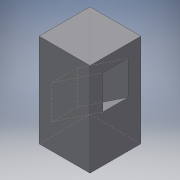
# Autodesk Inventor part: hollow monitor support (for assembly)
Saved by Autodesk Inventor 2016 (Build 200138000, 138)
## iProperties
Created: 2017-10-26
Part Number: hollow monitor support (for assembly)
Material: Generic
Document SubType Name: Modeling
Designer: student
Density: 1 g/cm^3
Appearance: Default
Author: student
Autodesk Inventor part; units mm, degrees
ref_plane "YZ Plane" through (0, 0, 0) normal (1, 0, 0) x (0, 1, 0)
ref_plane "XZ Plane" through (0, 0, 0) normal (0, 1, 0) x (-1, 0, 0)
ref_plane "XY Plane" through (0, 0, 0) normal (0, 0, 1) x (1, 0, 0)
sketch "Sketch1" plane through (0, 0, 0) normal (0, 0, 1) x (1, 0, 0)
  line L0 (-38.1, -69.85) -> (38.1, -69.85)
  line L1 (38.1, -69.85) -> (38.1, 69.85)
  line L2 (38.1, 69.85) -> (-38.1, 69.85)
  line L3 (-38.1, 69.85) -> (-38.1, -69.85)
  line L4 (38.1, 6.35) -> (-38.1, -57.15)
  line L5 (38.1, 57.15) -> (-38.1, -6.35)
  point P0 (0, 0)
  dimension "d0" = 139.7
  dimension "d1" = 76.2
  dimension "d2" = 76.2
  dimension "d3" = 12.7
  dimension "d5" = 12.7
  dimension "d12" = 76.2
  constraints: 12 end point, 4 point on line, 2 parallel, 1 horizontal, 1 perpendicular
  measures "d0" distance of L0.end L1.end
  measures "d1" distance of L0.start L0.end
  measures "d2" distance of L0.end L4.start
  measures "d3" distance of L0.start L4.end
  measures "d5" distance of L1.end L5.start
  measures "d12" distance from line of L2 L5.end
extrude "Extrusion1" add sketch "Sketch1" along normal blind 38.1 contours L3 L4 L1 L0 | L3 L2 L1 L5
sketch "Sketch2" plane through (0, 0, 38.1) normal (0, 0, 1) x (1, 0, 0)
  line L0 (-38.1, 69.85) -> (-38.1, -69.85) projected
  line L1 (38.1, -69.85) -> (-38.1, -69.85)
  line L2 (-38.1, -69.85) -> (-38.1, 69.85)
  line L3 (-38.1, 69.85) -> (38.1, 69.85)
  line L4 (38.1, 69.85) -> (38.1, -69.85)
  line L5 (38.1, -69.85) -> (-38.1, 69.85) construction
  line L6 (-38.1, -69.85) -> (38.1, 69.85) construction
  point P0 (0, 0)
  point P1 (-38.1, 0)
  constraints: 12 end point, 2 midpoint, 2 parallel, 1 horizontal, 1 perpendicular
extrude "Extrusion2" add sketch "Sketch2" along normal blind 19.05
sketch "Sketch3" plane through (0, 0, 0) normal (0, 0, -1) x (-1, 0, 0)
  line L0 (38.1, 69.85) -> (38.1, -69.85) projected
  line L1 (-38.1, -69.85) -> (38.1, -69.85)
  line L2 (38.1, -69.85) -> (38.1, 69.85)
  line L3 (38.1, 69.85) -> (-38.1, 69.85)
  line L4 (-38.1, 69.85) -> (-38.1, -69.85)
  line L5 (-38.1, -69.85) -> (38.1, 69.85) construction
  line L6 (38.1, -69.85) -> (-38.1, 69.85) construction
  point P0 (0, 0)
  point P1 (38.1, 0)
  constraints: 12 end point, 2 midpoint, 2 parallel, 1 horizontal, 1 perpendicular
extrude "Extrusion3" add sketch "Sketch3" along normal blind 19.05
body "Solid1"
